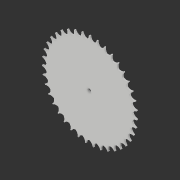
# Autodesk Inventor part: Sprocket Chain Positioning 2
Saved by Autodesk Inventor 2019 (Build 230136000, 136)
## iProperties
Created: 2020-06-02
Part Number: Sprocket Chain Positioning 2
Material: Generic
Document SubType Name: Modeling
Designer: 18186
Density: 1 g/cm^3
Appearance: Default
Author: 18186
Autodesk Inventor part; units mm, degrees
ref_plane "YZ Plane" through (0, 0, 0) normal (1, 0, 0) x (0, 1, 0)
ref_plane "XZ Plane" through (0, 0, 0) normal (0, 1, 0) x (-1, 0, 0)
ref_plane "XY Plane" through (0, 0, 0) normal (0, 0, 1) x (1, 0, 0)
sketch "Sketch1" plane through (0, 0, 0) normal (0, 0, 1) x (1, 0, 0)
  line L0 (-0.0002, 46.6475) -> (-0.0002, 89.1817) construction
  line L1 (-0.6352, 88.9) -> (0.6348, 88.9)
  arc A0 (0.6348, 88.9) -> (6.411, 80.3132) centre (9.9054, 88.9) ccw
  arc A1 (-6.4105, 80.3133) -> (-0.6352, 88.9) centre (-9.9062, 88.9) ccw
  arc A2 (-19.2107, 78.2449) -> (-14.8875, 87.6469) centre (-24.0385, 86.1597) ccw
  line L2 (-14.8875, 87.6469) -> (-13.634, 87.8506)
  arc A3 (-13.634, 87.8506) -> (-6.5552, 80.3016) centre (-4.4835, 89.3377) ccw
  arc A4 (-31.5133, 74.1501) -> (-28.7543, 84.1237) centre (-37.5482, 81.1879) ccw
  line L3 (-28.7543, 84.1237) -> (-27.5496, 84.5259)
  arc A5 (-27.5496, 84.5259) -> (-19.3516, 78.2102) centre (-18.7562, 87.4616) ccw
  arc A6 (-42.9997, 68.1347) -> (-41.8763, 78.4219) centre (-50.0854, 74.1134) ccw
  line L4 (-41.8763, 78.4219) -> (-40.7518, 79.0121)
  arc A7 (-40.7518, 79.0121) -> (-31.6468, 74.0932) centre (-32.5431, 83.3203) ccw
  arc A8 (-53.3724, 60.3548) -> (-53.9138, 70.6889) centre (-61.3254, 65.1194) ccw
  line L5 (-53.9138, 70.6889) -> (-52.8985, 71.4518)
  arc A9 (-52.8985, 71.4518) -> (-43.1223, 68.0572) centre (-45.4872, 77.021) ccw
  arc A10 (-62.3629, 51.0117) -> (-64.5549, 61.1251) centre (-70.9772, 54.4388) ccw
  line L6 (-64.5549, 61.1251) -> (-63.6751, 62.041)
  arc A11 (-63.6751, 62.041) -> (-53.4811, 60.2585) centre (-57.2532, 68.727) ccw
  arc A12 (-69.7381, 40.3474) -> (-73.5241, 49.9782) centre (-78.7906, 42.3483) ccw
  line L7 (-73.5241, 49.9782) -> (-72.8026, 51.0234)
  arc A13 (-72.8026, 51.0234) -> (-62.4546, 50.8992) centre (-67.5364, 58.6529) ccw
  arc A14 (-75.3072, 28.6381) -> (-80.589, 37.5369) centre (-84.5635, 29.161) ccw
  line L8 (-80.589, 37.5369) -> (-80.0446, 38.6843)
  arc A15 (-80.0446, 38.6843) -> (-69.8107, 40.2217) centre (-76.0704, 47.0598) ccw
  arc A16 (-78.9259, 16.1871) -> (-85.5668, 24.1234) centre (-88.1461, 15.2185) ccw
  line L9 (-85.5668, 24.1234) -> (-85.2134, 25.3433)
  arc A17 (-85.2134, 25.3433) -> (-75.3587, 28.5024) centre (-82.6342, 34.2478) ccw
  arc A18 (-80.5004, 3.3169) -> (-88.3284, 10.0852) centre (-89.4459, 0.8818) ccw
  line L10 (-88.3284, 10.0852) -> (-88.1753, 11.3459)
  arc A19 (-88.1753, 11.3459) -> (-78.9549, 16.0449) centre (-87.0579, 20.5489) ccw
  arc A20 (-79.99, -9.6392) -> (-88.8023, -4.2143) centre (-88.429, -13.4778) ccw
  line L11 (-88.8023, -4.2143) -> (-88.8535, -2.9453)
  arc A21 (-88.8535, -2.9453) -> (-80.5062, 3.1719) centre (-89.2268, 6.3177) ccw
  arc A22 (-77.4079, -22.3457) -> (-86.9763, -18.4046) centre (-85.1219, -27.4883) ccw
  line L12 (-86.9763, -18.4046) -> (-87.2304, -17.1603)
  arc A23 (-87.2304, -17.1603) -> (-79.9725, -9.7833) centre (-89.0847, -8.0771) ccw
  arc A24 (-72.821, -34.4734) -> (-82.8977, -32.1183) centre (-79.6102, -40.7868) ccw
  line L13 (-82.8977, -32.1183) -> (-83.3481, -30.9308)
  arc A25 (-83.3481, -30.9308) -> (-77.3675, -22.4851) centre (-86.6354, -22.2627) ccw
  arc A26 (-66.3481, -45.7083) -> (-76.6721, -45.0001) centre (-72.0366, -53.029) ccw
  line L14 (-76.6721, -45.0001) -> (-77.3071, -43.9002)
  arc A27 (-77.3071, -43.9002) -> (-72.7588, -34.6045) centre (-81.9423, -35.8717) ccw
  arc A28 (-58.1567, -55.7594) -> (-68.4607, -56.7164) centre (-62.5973, -63.8978) ccw
  line L15 (-68.4607, -56.7164) -> (-69.2639, -55.7327)
  arc A29 (-69.2639, -55.7327) -> (-66.2656, -45.8278) centre (-75.127, -48.5516) ccw
  arc A30 (-48.4592, -64.3663) -> (-58.4762, -66.9638) centre (-51.5367, -73.1116) ccw
  line L16 (-58.4762, -66.9638) -> (-59.4268, -66.1216)
  arc A31 (-59.4268, -66.1216) -> (-58.0562, -55.8641) centre (-66.3659, -59.9741) ccw
  arc A32 (-37.5066, -71.3062) -> (-46.9772, -75.4769) centre (-39.1414, -80.4319) ccw
  line L17 (-46.9772, -75.4769) -> (-48.0506, -74.7981)
  arc A33 (-48.0506, -74.7981) -> (-48.3432, -64.4535) centre (-55.8859, -69.8433) ccw
  arc A34 (-25.5826, -76.3993) -> (-34.2615, -82.0351) centre (-25.7323, -85.6691) ccw
  line L18 (-34.2615, -82.0351) -> (-35.4298, -81.5373)
  arc A35 (-35.4298, -81.5373) -> (-37.3781, -71.3736) centre (-43.9586, -77.9036) ccw
  arc A36 (-12.996, -79.5137) -> (-20.6584, -86.4687) centre (-11.6568, -88.6874) ccw
  line L19 (-20.6584, -86.4687) -> (-21.8915, -86.1648)
  arc A37 (-21.8915, -86.1648) -> (-25.4449, -76.4452) centre (-30.8927, -83.9462) ccw
  arc A38 (-0.0728, -80.5687) -> (-6.5204, -88.6628) centre (2.7206, -89.4088) ccw
  line L20 (-6.5204, -88.6628) -> (-7.7862, -88.5606)
  arc A39 (-7.7862, -88.5606) -> (-12.8527, -79.5369) centre (-17.0267, -87.8147) ccw
  arc A40 (12.8523, -79.537) -> (7.7866, -88.5606) centre (17.0275, -87.8146) ccw
  line L21 (7.7866, -88.5606) -> (6.5207, -88.6628)
  arc A41 (6.5207, -88.6628) -> (0.0723, -80.5687) centre (-2.7198, -89.4088) ccw
  arc A42 (25.4445, -76.4454) -> (21.8919, -86.1647) centre (30.8935, -83.946) ccw
  line L22 (21.8919, -86.1647) -> (20.6588, -86.4686)
  arc A43 (20.6588, -86.4686) -> (12.9955, -79.5137) centre (11.6576, -88.6872) ccw
  arc A44 (37.3777, -71.3738) -> (35.4302, -81.5372) centre (43.9593, -77.9033) ccw
  line L23 (35.4302, -81.5372) -> (34.2618, -82.035)
  arc A45 (34.2618, -82.035) -> (25.5821, -76.3994) centre (25.7331, -85.6688) ccw
  arc A46 (48.3428, -64.4538) -> (48.0509, -74.7979) centre (55.8866, -69.8429) ccw
  line L24 (48.0509, -74.7979) -> (46.9775, -75.4767)
  arc A47 (46.9775, -75.4767) -> (37.5062, -71.3064) centre (39.1421, -80.4315) ccw
  arc A48 (58.0559, -55.8644) -> (59.427, -66.1214) centre (66.3665, -59.9736) ccw
  line L25 (59.427, -66.1214) -> (58.4764, -66.9636)
  arc A49 (58.4764, -66.9636) -> (48.4588, -64.3666) centre (51.5373, -73.1111) ccw
  arc A50 (66.2654, -45.8281) -> (69.2641, -55.7324) centre (75.1275, -48.551) ccw
  line L26 (69.2641, -55.7324) -> (68.4609, -56.7161)
  arc A51 (68.4609, -56.7161) -> (58.1564, -55.7597) centre (62.5978, -63.8972) ccw
  arc A52 (72.7586, -34.6049) -> (77.3073, -43.8999) centre (81.9428, -35.871) ccw
  line L27 (77.3073, -43.8999) -> (76.6723, -44.9998)
  arc A53 (76.6723, -44.9998) -> (66.3478, -45.7087) centre (72.037, -53.0283) ccw
  arc A54 (77.3674, -22.4855) -> (83.3482, -30.9305) centre (86.6357, -22.2619) ccw
  line L28 (83.3482, -30.9305) -> (82.8978, -32.1179)
  arc A55 (82.8978, -32.1179) -> (72.8208, -34.4738) centre (79.6104, -40.7861) ccw
  arc A56 (79.9725, -9.7837) -> (87.2304, -17.1599) centre (89.0849, -8.0763) ccw
  line L29 (87.2304, -17.1599) -> (86.9764, -18.4043)
  arc A57 (86.9764, -18.4043) -> (77.4078, -22.3461) centre (85.1221, -27.4875) ccw
  arc A58 (80.5063, 3.1714) -> (88.8535, -2.945) centre (89.2268, 6.3185) ccw
  line L30 (88.8535, -2.945) -> (88.8023, -4.2139)
  arc A59 (88.8023, -4.2139) -> (79.99, -9.6397) centre (88.4291, -13.477) ccw
  arc A60 (78.955, 16.0445) -> (88.1753, 11.3463) centre (87.0578, 20.5497) ccw
  line L31 (88.1753, 11.3463) -> (88.3283, 10.0855)
  arc A61 (88.3283, 10.0855) -> (80.5004, 3.3165) centre (89.4458, 0.8826) ccw
  arc A62 (75.3588, 28.502) -> (85.2133, 25.3436) centre (82.634, 34.2486) ccw
  line L32 (85.2133, 25.3436) -> (85.5667, 24.1238)
  arc A63 (85.5667, 24.1238) -> (78.926, 16.1867) centre (88.1459, 15.2192) ccw
  arc A64 (69.8109, 40.2213) -> (80.0444, 38.6846) centre (76.07, 47.0605) ccw
  line L33 (80.0444, 38.6846) -> (80.5889, 37.5372)
  arc A65 (80.5889, 37.5372) -> (75.3074, 28.6377) centre (84.5631, 29.1617) ccw
  arc A66 (62.4549, 50.8989) -> (72.8024, 51.0237) centre (67.5359, 58.6536) ccw
  line L34 (72.8024, 51.0237) -> (73.5239, 49.9785)
  arc A67 (73.5239, 49.9785) -> (69.7383, 40.347) centre (78.7902, 42.349) ccw
  arc A68 (53.4814, 60.2583) -> (63.6749, 62.0413) centre (57.2526, 68.7276) ccw
  line L35 (63.6749, 62.0413) -> (64.5547, 61.1254)
  arc A69 (64.5547, 61.1254) -> (62.3631, 51.0113) centre (70.9766, 54.4394) ccw
  arc A70 (43.1227, 68.0569) -> (52.8982, 71.452) centre (45.4866, 77.0215) ccw
  line L36 (52.8982, 71.452) -> (53.9135, 70.6891)
  arc A71 (53.9135, 70.6891) -> (53.3728, 60.3545) centre (61.3248, 65.1199) ccw
  arc A72 (31.6472, 74.093) -> (40.7515, 79.0122) centre (32.5424, 83.3207) ccw
  line L37 (40.7515, 79.0122) -> (41.876, 78.422)
  arc A73 (41.876, 78.422) -> (43.0001, 68.1345) centre (50.0847, 74.1138) ccw
  arc A74 (19.352, 78.2101) -> (27.5493, 84.526) centre (18.7554, 87.4619) ccw
  line L38 (27.5493, 84.526) -> (28.7539, 84.1239)
  arc A75 (28.7539, 84.1239) -> (31.5137, 74.1499) centre (37.5474, 81.1882) ccw
  arc A76 (6.5556, 80.3016) -> (13.6336, 87.8507) centre (4.4827, 89.3378) ccw
  line L39 (13.6336, 87.8507) -> (14.8872, 87.6469)
  arc A77 (14.8872, 87.6469) -> (19.2111, 78.2448) centre (24.0377, 86.1598) ccw
  arc A78 (6.5556, 80.3016) -> (6.411, 80.3132) centre (0, 0) ccw
  arc A79 (19.352, 78.2101) -> (19.2111, 78.2448) centre (0, 0) ccw
  arc A80 (31.6472, 74.093) -> (31.5137, 74.1499) centre (0, 0) ccw
  arc A81 (-6.4105, 80.3133) -> (-6.5552, 80.3016) centre (0, 0) ccw
  arc A82 (-19.2107, 78.2449) -> (-19.3516, 78.2102) centre (0, 0) ccw
  arc A83 (-31.5133, 74.1501) -> (-31.6468, 74.0932) centre (0, 0) ccw
  arc A84 (-42.9997, 68.1347) -> (-43.1223, 68.0572) centre (0, 0) ccw
  arc A85 (-53.3724, 60.3548) -> (-53.4811, 60.2585) centre (0, 0) ccw
  arc A86 (-62.3629, 51.0117) -> (-62.4546, 50.8992) centre (0, 0) ccw
  arc A87 (-69.7381, 40.3474) -> (-69.8107, 40.2217) centre (0, 0) ccw
  arc A88 (-75.3072, 28.6381) -> (-75.3587, 28.5024) centre (0, 0) ccw
  arc A89 (-78.9259, 16.1871) -> (-78.9549, 16.0449) centre (0, 0) ccw
  arc A90 (-80.5004, 3.3169) -> (-80.5062, 3.1719) centre (0, 0) ccw
  arc A91 (-79.99, -9.6392) -> (-79.9725, -9.7833) centre (0, 0) ccw
  arc A92 (-77.4079, -22.3457) -> (-77.3675, -22.4851) centre (0, 0) ccw
  arc A93 (-72.821, -34.4734) -> (-72.7588, -34.6045) centre (0, 0) ccw
  arc A94 (-66.3481, -45.7083) -> (-66.2656, -45.8278) centre (0, 0) ccw
  arc A95 (-58.1567, -55.7594) -> (-58.0562, -55.8641) centre (0, 0) ccw
  arc A96 (-48.4592, -64.3663) -> (-48.3432, -64.4535) centre (0, 0) ccw
  arc A97 (-37.5066, -71.3062) -> (-37.3781, -71.3736) centre (0, 0) ccw
  arc A98 (-25.5826, -76.3993) -> (-25.4449, -76.4452) centre (0, 0) ccw
  arc A99 (-12.996, -79.5137) -> (-12.8527, -79.5369) centre (0, 0) ccw
  arc A100 (-0.0728, -80.5687) -> (0.0723, -80.5687) centre (0, 0) ccw
  arc A101 (12.8523, -79.537) -> (12.9955, -79.5137) centre (0, 0) ccw
  arc A102 (25.4445, -76.4454) -> (25.5821, -76.3994) centre (0, 0) ccw
  arc A103 (37.3777, -71.3738) -> (37.5062, -71.3064) centre (0, 0) ccw
  arc A104 (48.3428, -64.4538) -> (48.4588, -64.3666) centre (0, 0) ccw
  arc A105 (58.0559, -55.8644) -> (58.1564, -55.7597) centre (0, 0) ccw
  arc A106 (77.3674, -22.4855) -> (77.4078, -22.3461) centre (0, 0) ccw
  arc A107 (66.2654, -45.8281) -> (66.3478, -45.7087) centre (0, 0) ccw
  arc A108 (72.7586, -34.6049) -> (72.8208, -34.4738) centre (0, 0) ccw
  arc A109 (79.9725, -9.7837) -> (79.99, -9.6397) centre (0, 0) ccw
  arc A110 (80.5063, 3.1714) -> (80.5004, 3.3165) centre (0, 0) ccw
  arc A111 (78.955, 16.0445) -> (78.926, 16.1867) centre (0, 0) ccw
  arc A112 (43.1227, 68.0569) -> (43.0001, 68.1345) centre (0, 0) ccw
  arc A113 (53.4814, 60.2583) -> (53.3728, 60.3545) centre (0, 0) ccw
  arc A114 (62.4549, 50.8989) -> (62.3631, 51.0113) centre (0, 0) ccw
  arc A115 (75.3588, 28.502) -> (75.3074, 28.6377) centre (0, 0) ccw
  arc A116 (69.8109, 40.2213) -> (69.7383, 40.347) centre (0, 0) ccw
  circle A117 centre (0, 0) radius 80.5687 construction
  dimension "d17" = 161.1374
  dimension "d2" = 1.27
  dimension "d3" = 0.635
  dimension "d4" = 9.2706
  dimension "d5" = 9.271
  dimension "d6" = 360
  dimension "d8" = 0.1409
  dimension "d9" = 0.0347
  dimension "d16" = 88.9
  constraints: 156 point on circle, 80 end point, 78 centre point, 2 line through centre, 1 coincident, 1 horizontal, 1 horizontal alignment, 1 vertical, 473 other
  measures "d2" distance of L1.start L1.end
  measures "d3" distance from line of L1.end L0
  measures "d4" radius of A0
  measures "d5" radius of A1
  measures "d8" horizontal distance of A74.start A77.end
  measures "d9" vertical distance of A74.start A77.end
  measures "d16" distance from line of point (0, 0) L1
extrude "Extrusion1" add sketch "Sketch1" along normal blind 2.54
sketch "Sketch2" plane through (0, 0, 2.54) normal (0, 0, 1) x (1, 0, 0)
  circle A0 centre (0, 0) radius 3.175
  dimension "d12" = 6.35
  constraints: 1 centre point, 1 coincident
  measures "d12" diameter of A0
extrude "Extrusion2" cut sketch "Sketch2" against normal blind 25.4
body "Solid1"
